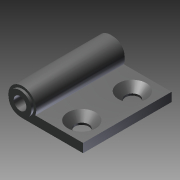
# Autodesk Inventor part: HHPFRN5-2
Saved by Autodesk Inventor 2011 SP1 (Build 150282100, 282)
## iProperties
Created: 2017-04-19
Part Number: HHPFRN5-2
Catalog Web Link: www.cadenas.de
Description: HHPFLN, HHPFRN-2-Aluminum Flag Hinges
Vendor: MISUMI
Document SubType Name: Modeling
Designer: psAdmin
Manufacturer: MISUMI
Mass: 4.86234 g
Surface Area: 35.1362 cm^2
Volume: 4.86234 cm^3
Density: 1 g/cm^3
Category: PARTsolutions
Company: MISUMI
Title: HHPFRN5-2
Author: Cadenas PARTsolutions
Comments: Aluminum Flag Hinges
PSOL_IDENT_0: {$CADENAS_DATA\23d-libs\misumi\metric\39_accessories_for_al_extrusions\hhpfln_2.prj},177 {VTYP=3D},{
PSOL_IDENT_1: NB=HHPFRN5-2},{LINA=HHPFRN5-2},{NN=HHPFLN, HHPFRN-2},{DATE=17.06.2016 05:53:44},{GEOMDATE=07.05.2009
PSOL_IDENT_2: 08:36:00},{VERSION=},{LINEID=10},{LINESUBID=-1},{WBVAR=TS,ALT1}  {NB=HHPFRN5-2},{LINA=HHPFRN5-2},{K
PSOL_IDENT_3: T=DUMMY},{PN=HHPFRN5},{TYPE=HHPFRN},{TS=HHPFRN},{MAT=6063 Aluminum Bushing - Polyacetal},{ST=Anodizi
PSOL_IDENT_4: ng},{NO=5},{ALKG=10},{ALN=98},{MASS=36},{L=35},{W=48},{K=7.5},{P=20},{J=8.0},{F=16.0},{V=10.5},{ND=5
PSOL_IDENT_5: .5},{NC=11},{T=3.5},{Y=38.5},{AB=FB5-8},{QB=4},{AN=HNTT5-5},{QN=4},{ALT1=}
NN: HHPFLN, HHPFRN-2
NT: Aluminum Flag Hinges
NB: HHPFRN5-2
NBSYN: $PN.-2
LINA: HHPFRN5-2
TS: For Right-Hand Use
MAT: 6063 Aluminum Bushing - Polyacetal
ST: Anodizing
NO: 5
ALKG: 10
ALN: 98
MASS: 36
L: 35
W: 48
K: 7.5
P: 20
J: 8.0
F: 16.0
V: 10.5
ND: 5.5
NC: 11
T: 3.5
Y: 38.5
AB: FB5-8
QB: 4
AN: HNTT5-5
QN: 4
ALT1: w/o Set of Applicable Bolt and Nut
SUPPLIER: MISUMI
ARTICLENO: HHPFRN5-2
BOMINFO: HHPFRN5-2
CREATOR: CADENAS GmbH
Autodesk Inventor part; units mm, degrees
sketch "Sketch_1" plane through (0, 0, 0) normal (0, 0, 1) x (1, 0, 0)
  line L0 (0, 0) -> (0, 36.8)
  line L1 (0, 36.8) -> (4.5, 36.8)
  line L2 (4.5, 36.8) -> (4.5, 35.9)
  line L3 (4.5, 35.9) -> (5.5, 35.9)
  line L4 (5.5, 35.9) -> (5.5, 0.9)
  line L5 (5.5, 0.9) -> (4.5, 0.9)
  line L6 (4.5, 0.9) -> (4.5, 0)
  line L7 (4.5, 0) -> (0, 0)
  line L8 (0, 0) -> (0, 36.8)
  constraints: 18 end point
revolve "Revolution1" add sketch "Sketch_1" angle 360 about axis through (0, 0, 0) along (0, -1, 0)
sketch "Sketch_3" plane through (0, 0, -5.5) normal (0, 0, 1) x (1, 0, 0)
  line L0 (0, 35.9) -> (0, 0.9)
  line L1 (0, 0.9) -> (24, 0.9)
  line L2 (24, 0.9) -> (24, 35.9)
  line L3 (24, 35.9) -> (0, 35.9)
  constraints: 8 end point
extrude "Extrusion1" add sketch "Sketch_3" along normal blind 3.5
sketch "Sketch3" plane through (0, 0, -2) normal (0, 0, 1) x (1, 0, 0)
  point P0 (16, 8.4)
hole "Hole1" at (16, 8.4, -2) direction (0, 0, -1) diameter 5.5 depth 3.5 countersink diameter 11 countersink angle 90
sketch "Sketch4" plane through (0, 0, -2) normal (0, 0, 1) x (1, 0, 0)
  point P0 (16, 28.4)
hole "Hole2" at (16, 28.4, -2) direction (0, 0, -1) diameter 5.5 depth 3.5 countersink diameter 11 countersink angle 90
sketch "Sketch5" plane through (0, 0, 0) normal (0, -1, 0) x (1, 0, 0)
  point P0 (0, 0)
hole "Hole3" at (0, 0, 0) direction (0, 1, 0) diameter 5 depth 36.8
ref_plane "2_XY" through (0, 0, 0) normal (0, 1, 0) x (1, 0, 0)
ref_plane "2_YZ" through (0, 0, 0) normal (1, 0, 0) x (0, 0, -1)
ref_plane "2_ZX" through (0, 0, 0) normal (0, 0, -1) x (0, 1, 0)
ref_plane "to_bolt3_XY" through (-16, 28.4, -2) normal (0, 0, 1) x (1, 0, 0)
ref_plane "to_bolt3_YZ" through (-16, 28.4, -2) normal (1, 0, 0) x (0, 1, 0)
ref_plane "to_bolt3_ZX" through (-16, 28.4, -2) normal (0, 1, 0) x (0, 0, 1)
ref_plane "to_bolt3_r_XY" through (16, 28.4, -2) normal (0, 0, 1) x (1, 0, 0)
ref_plane "to_bolt3_r_YZ" through (16, 28.4, -2) normal (1, 0, 0) x (0, 1, 0)
ref_plane "to_bolt3_r_ZX" through (16, 28.4, -2) normal (0, 1, 0) x (0, 0, 1)
ref_plane "to_bolt4_XY" through (-16, 8.4, -2) normal (0, 0, 1) x (1, 0, 0)
ref_plane "to_bolt4_YZ" through (-16, 8.4, -2) normal (1, 0, 0) x (0, 1, 0)
ref_plane "to_bolt4_ZX" through (-16, 8.4, -2) normal (0, 1, 0) x (0, 0, 1)
ref_plane "to_bolt4_r_XY" through (16, 8.4, -2) normal (0, 0, 1) x (1, 0, 0)
ref_plane "to_bolt4_r_YZ" through (16, 8.4, -2) normal (1, 0, 0) x (0, 1, 0)
ref_plane "to_bolt4_r_ZX" through (16, 8.4, -2) normal (0, 1, 0) x (0, 0, 1)
body "Solid1"
